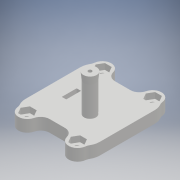
# Autodesk Inventor part: DAQcapsule_v2Top
Saved by Autodesk Inventor 2018 (Build 220112000, 112)
## iProperties
Created: 2020-03-10
Part Number: DAQcapsule_v2Top
Material: Generic
Document SubType Name: Modeling
Designer: Ivan
Density: 1 g/cm^3
Appearance: Default
Author: Ivan
Autodesk Inventor part; units mm, degrees
ref_plane "YZ Plane" through (0, 0, 0) normal (1, 0, 0) x (0, 1, 0)
ref_plane "XZ Plane" through (0, 0, 0) normal (0, 1, 0) x (-1, 0, 0)
ref_plane "XY Plane" through (0, 0, 0) normal (0, 0, 1) x (1, 0, 0)
sketch "Sketch1" plane through (0, 0, 0) normal (0, 0, 1) x (1, 0, 0)
  line L0 (-12.5, 11) -> (12.5, 11)
  line L1 (12.5, 11) -> (12.5, -11)
  line L2 (12.5, -11) -> (-12.5, -11)
  line L3 (-12.5, -11) -> (-12.5, 11)
  point P0 (0, 0)
  point P1 (0, 11)
  point P2 (-12.5, 0)
  dimension "d0" = 25
  dimension "d1" = 22
  constraints: 8 end point, 2 midpoint, 2 parallel, 1 horizontal, 1 horizontal alignment, 1 perpendicular, 1 vertical alignment
  measures "d0" distance of L0.start L0.end
  measures "d1" distance of L2.end L0.start
extrude "Extrusion1" add sketch "Sketch1" along normal blind 4
sketch "Sketch2" plane through (0, 0, 4) normal (0, 0, 1) x (1, 0, 0)
  circle A0 centre (8.45, -12.62) radius 3
  line L0 (12.5, -11) -> (-12.5, -11) construction
  circle A1 centre (8.45, -12.62) radius 1.05
  line L1 (-12.5, -11) -> (12.5, -11) construction
  line L2 (0, -11) -> (0, 11) construction
  line L3 (12.5, 11) -> (-12.5, 11) construction
  line L4 (-12.5, 0) -> (12.5, 0) construction
  line L5 (12.5, -11) -> (12.5, 11) construction
  circle A2 centre (-8.45, -12.62) radius 3
  circle A3 centre (-8.45, -12.62) radius 1.05
  circle A4 centre (8.45, 12.62) radius 3
  circle A5 centre (8.45, 12.62) radius 1.05
  circle A6 centre (-8.45, 12.62) radius 3
  circle A7 centre (-8.45, 12.62) radius 1.05
  point P0 (0, 0)
  dimension "d4" = 6
  dimension "d5" = 2.1
  dimension "d6" = 4.05
  dimension "d7" = 1.62
  constraints: 8 centre point, 6 end point, 6 symmetric about line, 4 coincident, 3 midpoint, 6 other
  measures "d4" diameter of A0
  measures "d5" diameter of A1
  measures "d6" horizontal distance of L0.start A0.centre
  measures "d7" distance from line of A0.centre L0
sketch "Sketch3" plane through (0, 0, 4) normal (0, 0, 1) x (1, 0, 0)
  line L0 (12.5, -11) -> (12.5, 11) construction
  line L1 (-12.5, -11) -> (12.5, -11) construction
  circle A0 centre (2.75, -2.75) radius 2
  point P0 (0, 0)
  point P1 (11.0064, -11)
  dimension "d10" = 4
  dimension "d11" = 9.75
  dimension "d12" = 8.25
  constraints: 1 centre point
  measures "d10" diameter of A0
  measures "d11" distance from line of L0 A0.centre
  measures "d12" distance from line of L1 A0.centre
extrude "Extrusion3" add sketch "Sketch3" along normal blind 10
sketch "Sketch6" plane through (0, 0, 4) normal (0, 0, 1) x (1, 0, 0)
  line L0 (-7, 2.5) -> (-5.5, 2.5)
  line L1 (-5.5, 2.5) -> (-5.5, -2.5)
  line L2 (-5.5, -2.5) -> (-7, -2.5)
  line L3 (-7, -2.5) -> (-7, 2.5)
  line L4 (-12.5, 11) -> (-12.5, -11) projected
  point P0 (0, 0)
  point P1 (-7, 0)
  point P2 (-12.5, 0)
  dimension "d24" = 1.5
  dimension "d25" = 5
  dimension "d30" = 5.5
  constraints: 8 end point, 2 horizontal alignment, 2 parallel, 1 horizontal, 1 midpoint, 1 perpendicular
  measures "d24" distance of L1.end L2.end
  measures "d25" distance of L0.end L1.end
  measures "d30" distance between parallel lines of L4 L3
extrude "Extrusion5" cut sketch "Sketch6" against normal through all
extrude "Extrusion7" add sketch "Sketch2" against normal up to surface (4 mm away)
sketch "Sketch8" plane through (0, 0, 4) normal (0, 0, 1) x (1, 0, 0)
  circle A0 centre (8.45, -12.62) radius 1.05 construction
  line L0 (7.3, -10.6281) -> (9.6, -10.6281)
  line L1 (9.6, -10.6281) -> (10.75, -12.62)
  line L2 (10.75, -12.62) -> (9.6, -14.6119)
  line L3 (9.6, -14.6119) -> (7.3, -14.6119)
  line L4 (7.3, -14.6119) -> (6.15, -12.62)
  line L5 (6.15, -12.62) -> (7.3, -10.6281)
  line L6 (-5.925, -11) -> (5.925, -11) projected
  line L7 (0, -11) -> (0, 0) construction
  line L8 (-7.3, -10.6281) -> (-9.6, -10.6281)
  line L9 (-9.6, -10.6281) -> (-10.75, -12.62)
  line L10 (-10.75, -12.62) -> (-9.6, -14.6119)
  line L11 (-9.6, -14.6119) -> (-7.3, -14.6119)
  line L12 (-7.3, -14.6119) -> (-6.15, -12.62)
  line L13 (-6.15, -12.62) -> (-7.3, -10.6281)
  line L14 (12.5, -11) -> (12.5, 11) construction
  line L15 (12.5, 0) -> (0, 0) construction
  line L16 (7.3, 10.6281) -> (9.6, 10.6281)
  line L17 (9.6, 10.6281) -> (10.75, 12.62)
  line L18 (10.75, 12.62) -> (9.6, 14.6119)
  line L19 (9.6, 14.6119) -> (7.3, 14.6119)
  line L20 (7.3, 14.6119) -> (6.15, 12.62)
  line L21 (6.15, 12.62) -> (7.3, 10.6281)
  line L22 (-7.3, 14.6119) -> (-6.15, 12.62)
  line L23 (-9.6, 14.6119) -> (-7.3, 14.6119)
  line L24 (-10.75, 12.62) -> (-9.6, 14.6119)
  line L25 (-9.6, 10.6281) -> (-10.75, 12.62)
  line L26 (-7.3, 10.6281) -> (-9.6, 10.6281)
  line L27 (-6.15, 12.62) -> (-7.3, 10.6281)
  dimension "d38" = 4.6
  constraints: 52 end point, 18 symmetric about line, 2 midpoint, 1 coincident, 1 parallel, 1 perpendicular, 1 vertical, 13 other
  measures "d38" distance of L4.end L1.end
extrude "Extrusion8" cut sketch "Sketch8" against normal blind 2
ref_plane "Work Plane2" through (2.75, -2.75, 16.5) normal (0, 0, 1) x (1, 0, 0)
sketch "Sketch9" plane through (2.75, -2.75, 16.5) normal (0, 0, 1) x (1, 0, 0)
  circle A0 centre (0, 0) radius 2.25
  point P0 (-2.75, 2.75)
  dimension "d42" = 4.5
  constraints: 1 centre point, 1 coincident
  measures "d42" diameter of A0
loft "Loft2" add profiles "Sketch9" section 2 edges at (0.75, -2.75, 14)
fillet "Fillet1" radius 3 8 edges at (5.925, 11, 2) (10.975, 11, 2) (-5.925, 11, 2) (-10.975, 11, 2) (-10.975, -11, 2) (-5.925, -11, 2) (5.925, -11, 2) (10.975, -11, 2)
fillet "Fillet2" radius 5 4 edges at (-12.5, -11, 2) (-12.5, 11, 2) (12.5, 11, 2) (12.5, -11, 2)
sketch "Sketch10" plane through (2.75, -2.75, 16.5) normal (0, 0, 1) x (1, 0, 0)
  circle A0 centre (0, 0) radius 2 construction
  circle A1 centre (0, 0) radius 0.625
  point P0 (-2.75, 2.75)
  dimension "d49" = 1.25
  constraints: 1 centre point, 1 coincident
  measures "d49" diameter of A1
extrude "Extrusion9" cut sketch "Sketch10" against normal up to surface (16.5 mm away)
equation "\"d6\" = 0.5 * d4 + 0.5 * d5"
equation "\"d7\" = 0.4 * d6"
body "Solid1"
